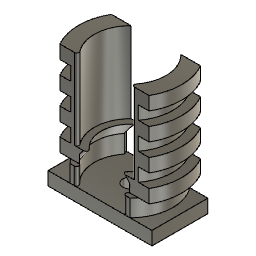
X_carriage_-_Cable_locker_JSR (Autodesk Fusion 360 design; units mm, degrees)
Autodesk Fusion 360 part; units mm, degrees
note: some values were not read from the file. Set by a fixed rule: which sketch regions a step uses.
sketch "Sketch1" plane through (0, 0, 0) normal (0, 0, 1) x (1, 0, 0)
  line L0 (11.6, -11.5) -> (-11.6, -11.5)
  line L1 (-11.6, -11.5) -> (-11.6, 11.5)
  line L2 (-11.6, 11.5) -> (11.6, 11.5)
  line L3 (11.6, 11.5) -> (11.6, -11.5)
  line L4 (11.6, -11.5) -> (-11.6, 11.5) construction
  line L5 (-11.6, -11.5) -> (11.6, 11.5) construction
  circle A0 centre (0, 0) radius 1.625
  dimension "d1" = 23.2
  dimension "d2" = 23
  dimension "d29" = 3.25
  constraint horizontal L0
  constraint perpendicular L0 L1
  constraint parallel L0 L2
  constraint parallel L1 L3
  constraint coincident L4 A0.centre
  constraint coincident L5 A0.centre
  constraint coincident A0.centre origin
  measures "d1" distance of L1.end L2.end
  measures "d2" distance of L0.end L1.end
  measures "d29" diameter of A0
extrude "Extrude2" add sketch "Sketch1" along normal blind 3 makes body 1
sketch "Sketch2" plane through (0, 0, 0) normal (0, 1, 0) x (1, 0, 0)
  line L0 (0, 0) -> (0, -3) construction
  line L1 (0, -3) -> (9.5, -3)
  line L2 (9.5, -3) -> (9.5, -6.8)
  line L3 (9.5, -6.8) -> (11.5, -6.8)
  line L4 (11.5, -6.8) -> (11.5, -9.8)
  line L5 (11.5, -9.8) -> (9.5, -9.8)
  line L6 (9.5, -9.8) -> (9.5, -12.8)
  line L7 (9.5, -12.8) -> (11.5, -12.8)
  line L8 (11.5, -12.8) -> (11.5, -15.8)
  line L9 (11.5, -15.8) -> (9.5, -15.8)
  line L10 (9.5, -15.8) -> (9.5, -18.8)
  line L11 (9.5, -18.8) -> (11.5, -18.8)
  line L12 (11.5, -18.8) -> (11.5, -21.8)
  line L13 (11.5, -21.8) -> (9.5, -21.8)
  line L14 (9.5, -21.8) -> (9.5, -24.8)
  line L15 (9.5, -24.8) -> (11.5, -24.8)
  line L16 (11.5, -24.8) -> (11.5, -27.8)
  line L17 (11.5, -27.8) -> (8, -27.8)
  line L18 (8, -27.8) -> (8, -9.8)
  line L19 (8, -9.8) -> (6.5, -9.8)
  line L20 (9.5, -3) -> (8, -3)
  line L21 (8, -3) -> (8, -7)
  line L22 (8, -7) -> (6.5, -9.8)
  dimension "d10" = 3
  dimension "d11" = 9.5
  dimension "d12" = 3.8
  dimension "d13" = 2
  dimension "d14" = 3
  dimension "d15" = 2
  dimension "d16" = 3
  dimension "d17" = 2
  dimension "d18" = 3
  dimension "d19" = 2
  dimension "d20" = 3
  dimension "d21" = 2
  dimension "d22" = 3
  dimension "d23" = 2
  dimension "d24" = 3
  dimension "d25" = 2
  dimension "d26" = 3
  dimension "d27" = 3.5
  dimension "d45" = 18
  dimension "d46" = 1.5
  dimension "d64" = 1.5
  dimension "d65" = 2.8
  constraint coincident L0.start origin
  constraint vertical L0
  constraint perpendicular L0 L1
  constraint perpendicular L1 L2
  constraint perpendicular L2 L3
  constraint perpendicular L3 L4
  constraint perpendicular L4 L5
  constraint perpendicular L5 L6
  constraint perpendicular L6 L7
  constraint perpendicular L7 L8
  constraint perpendicular L8 L9
  constraint perpendicular L9 L10
  constraint perpendicular L10 L11
  constraint perpendicular L11 L12
  constraint perpendicular L12 L13
  constraint perpendicular L13 L14
  constraint perpendicular L14 L15
  constraint perpendicular L15 L16
  constraint perpendicular L16 L17
  constraint perpendicular L17 L18
  constraint perpendicular L18 L19
  constraint coincident L1 L20.end
  constraint perpendicular L1 L21
  measures "d10" distance of L0.start L0.end
  measures "d11" distance of L0.end L1.end
  measures "d12" distance of L1.end L2.end
  measures "d13" distance of L2.end L3.end
  measures "d14" distance of L3.end L4.end
  measures "d15" distance of L4.end L5.end
  measures "d16" distance of L5.end L6.end
  measures "d17" distance of L6.end L7.end
  measures "d18" distance of L7.end L8.end
  measures "d19" distance of L8.end L9.end
  measures "d20" distance of L9.end L10.end
  measures "d21" distance of L10.end L11.end
  measures "d22" distance of L11.end L12.end
  measures "d23" distance of L12.end L13.end
  measures "d24" distance of L13.end L14.end
  measures "d25" distance of L14.end L15.end
  measures "d26" distance of L15.end L16.end
  measures "d27" distance of L16.end L17.end
  measures "d45" distance of L17.end L18.end
  measures "d46" distance of L18.end L19.end
  measures "d64" distance of L1.end L20.end
  measures "d65" vertical distance of L19.end L21.end
revolve "Revolve1" add sketch "Sketch2" angle 360 about axis through (0, 0, 1.75) along (0, 0, 1) makes body 2
sketch "Sketch3" plane through (0, 0, 0) normal (0, 0, 1) x (1, 0, 0)
  line L0 (0, 0) -> (-11.6, 0) construction
  line L1 (-11.6, 0) -> (-11.6, 5.75) construction
  line L2 (-11.6, 11.5) -> (-11.6, 5.75)
  line L3 (-11.6, 5.75) -> (11.6, 5.75)
  line L4 (11.6, 5.75) -> (11.6, 11.5)
  line L5 (11.6, 11.5) -> (-11.6, 11.5)
  line L6 (-11.6, 11.5) -> (-11.6, 5.75)
  line L7 (-11.6, 0) -> (-11.6, -6.75) construction
  line L8 (-11.6, -6.75) -> (11.6, -6.75)
  line L9 (11.6, -6.75) -> (11.6, -11.5)
  line L10 (11.6, -11.5) -> (-11.6, -11.5)
  line L11 (-11.6, -11.5) -> (-11.6, -6.75)
  dimension "d32" = 11.6
  dimension "d36" = 5.75
  dimension "d39" = 23.2
  dimension "d40" = 5.75
  dimension "d41" = 6.75
  dimension "d42" = 23.2
  dimension "d43" = 4.75
  constraint coincident L0.start origin
  constraint horizontal L0
  constraint perpendicular L0 L1
  constraint vertical L2
  constraint horizontal L3
  constraint vertical L4
  constraint horizontal L5
  constraint vertical L6
  constraint perpendicular L0 L7
  constraint horizontal L8
  constraint vertical L9
  constraint horizontal L10
  constraint vertical L11
  measures "d32" distance of L0.start L0.end
  measures "d36" distance of L0.end L1.end
  measures "d39" distance of L1.end L3.end
  measures "d40" distance of L1.end L2.start
  measures "d41" distance of L0.end L7.end
  measures "d42" distance of L7.end L8.end
  measures "d43" distance of L7.end L10.end
extrude "Extrude3" cut sketch "Sketch3" along normal through all bodies 1 2
sketch "Sketch5" plane through (0, 0, 6.8) normal (0, 0, -1) x (1, 0, 0)
  line L0 (-6.6849, 6.75) -> (-9.3106, 6.75)
  line L1 (-9.9593, -5.75) -> (-7.5622, -5.75)
  line L2 (0, 0) -> (0, 5.75) construction
  line L3 (0, 5.75) -> (-11.5, 5.75) construction
  line L4 (-11.5, 5.75) -> (11.5, 5.75)
  line L5 (11.5, 5.75) -> (11.5, 11.5)
  line L6 (11.5, 11.5) -> (-11.5, 11.5)
  line L7 (-11.5, 11.5) -> (-11.5, 5.75)
  dimension "d52" = 5.75
  dimension "d53" = 11.5
  dimension "d54" = 23
  dimension "d55" = 5.75
  constraint coincident L2.start origin
  constraint vertical L2
  constraint perpendicular L2 L3
  constraint horizontal L4
  constraint vertical L5
  constraint horizontal L6
  constraint vertical L7
  measures "d52" distance of L2.start L2.end
  measures "d53" distance of L2.end L3.end
  measures "d54" distance of L3.end L4.end
  measures "d55" distance of L3.end L6.end
extrude "Extrude4" cut sketch "Sketch5" against normal through all bodies 2 makes body 3 at (-5.835, -5.473, 21.8)
fillet "Fillet4" radius 0.5 6 edges at (4.2939, -6.75, 4.9) (4.1945, -5.75, 8.6477) (5.5621, -5.75, 18.8) (-4.2939, -6.75, 4.9) (-4.1945, -5.75, 8.6477) (-5.5621, -5.75, 18.8) on bodies 2 3
chamfer "Chamfer1" distance 1 angle 45 4 edges at (5.5621, 5.75, 5) (4.2307, 5.75, 8.6078) (-5.5621, 5.75, 5) (-4.2307, 5.75, 8.6078) on bodies 2 3
